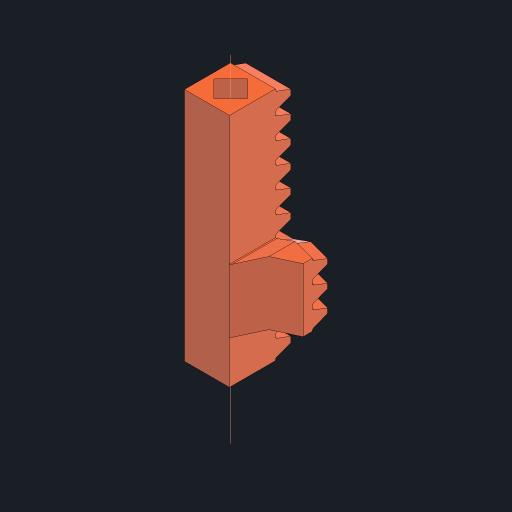
# Autodesk Inventor part: Rack V3
Saved by Autodesk Inventor 2023.2 (Build 272271030, 271C)
## iProperties
Created: 2023-11-19
Part Number: Rack V3
Material: Generic
Document SubType Name: Modeling
Designer: robpl
Density: 1 g/cm^3
Appearance: Smooth - Light Orange
Author: robpl
## iProperties of the stored document Rack_3DPrint.ipt
Created: 2023-11-27
Part Number: Rack_3DPrint
Material: Generic
Document SubType Name: Modeling
Designer: robpl
Density: 1 g/cm^3
Appearance: Default
Author: robpl
Autodesk Inventor part; units mm, degrees
ref_plane "YZ Plane" through (0, 0, 0) normal (1, 0, 0) x (0, 1, 0)
ref_plane "XZ Plane" through (0, 0, 0) normal (0, 1, 0) x (-1, 0, 0)
ref_plane "XY Plane" through (0, 0, 0) normal (0, 0, 1) x (1, 0, 0)
sketch "Sketch1" plane through (0, 0, 0) normal (0, 0, 1) x (1, 0, 0)
  line L0 (0, 0) -> (-12, 0)
  line L1 (-12, 0) -> (-12, 34.557519)
  line L2 (-12, 34.557519) -> (0, 34.557519)
  line L3 (0, 34.557519) -> (0, 0)
  dimension "d0" = 12
  dimension "d1" = 34.55752
  constraints: 8 end point, 2 parallel, 1 horizontal, 1 perpendicular
  measures "d0" distance of L1.end L2.end
  measures "d1" distance of L0.end L1.end
extrude "Extrusion1" add sketch "Sketch1" along normal blind 9
sketch "Sketch2" plane through (-12, 0, 0) normal (1, 0, 0) x (0, 0, -1)
  line L0 (0, 0) -> (0, 34.557519)
  line L1 (0, 34.557519) -> (-9, 34.557519)
  line L2 (-9, 0) -> (-9, 34.557519)
  line L3 (0, 0) -> (-9, 0)
  line L4 (0, 1.149368) -> (-2.25, 0.330435)
  line L5 (-2.25, 0.330435) -> (-2.25, -0.330435)
  line L6 (-2.25, -0.330435) -> (0, -1.149368)
  line L7 (0, -1.149368) -> (0, 1.149368)
  line L8 (-1, -0.785398) -> (-1, 0.785398)
  line L9 (0, 0) -> (-9, 0)
  arc A0 (-2.25, -0.064357) -> (-1.999968, -0.42144) centre (-1.87, -0.064357) ccw
  arc A1 (-1.999968, 0.42144) -> (-2.25, 0.064357) centre (-1.87, 0.064357) ccw
  point P0 (-2.25, 0)
  point P1 (0, 0)
  point P2 (-2.25, 0)
  dimension "d4" = 1
  dimension "d5" = 1.25
  dimension "d6" = 1.5708
  dimension "d7" = 70
  dimension "d17" = 0.38
  constraints: 10 end point, 8 point on line, 4 point on circle, 4 tangent, 3 vertical, 2 centre point, 1 equal length, 1 equal radius, 1 midpoint
  measures "d4" distance between parallel lines of L0 L8
  measures "d5" distance between parallel lines of L5 L8
  measures "d6" distance of L8.start L8.end
  measures "d7" angle of L6 L8
  measures "d17" radius of A0
sketch "Sketch3" plane through (0, 0, 0) normal (0, 0, -1) x (-1, 0, 0)
  line L0 (12, -1.149368) -> (12, 1.149368)
  line L1 (12, -1.149368) -> (5, -1.149368)
  line L2 (5, -1.149368) -> (2.5, -0.239443)
  line L3 (2.5, -0.239443) -> (0, -1.149368)
  point P0 (0, 0)
  dimension "d27" = 7
  dimension "d28" = 5
  dimension "d29" = 20
  constraints: 6 end point, 1 equal length, 1 horizontal, 1 point on line
  measures "d27" distance of L0.start L1.end
  measures "d28" distance of L1.end L3.end
  measures "d29" angle of L1 L2
sweep "Sweep1" cut profiles "Sketch2" path "Sketch3" path curves L1 L2 L3 contours L3 L8 L4 L0 | L7 L6 L8 L3 | L8 L6 A0 L5 L3 | L3 L5 A1 L4 L8
pattern_linear "Rectangular Pattern1" count 12 spacing 3.141593 along (0, 1, 0) of "Sweep1"
sketch "Sketch4" plane through (-12, 34.557519, 9) normal (0, 1, 0) x (1, 0, 0)
  line L0 (0, 6.75) -> (0, 0)
  line L1 (12, 0) -> (0, 0)
  line L2 (12, 6.750032) -> (12, 0)
  line L3 (3.3, 5.974874) -> (0.825126, 3.5)
  line L4 (0.825126, 3.5) -> (3.3, 1.025126)
  line L5 (3.3, 1.025126) -> (5.774874, 3.5)
  line L6 (5.774874, 3.5) -> (3.3, 5.974874)
  line L7 (3.3, 5.974874) -> (3.3, 1.025126) construction
  line L8 (0.825126, 3.5) -> (5.774874, 3.5) construction
  line L9 (0, 6.75) -> (0, 0)
  line L10 (0, 9) -> (7, 9)
  line L11 (10.970457, 7.000032) -> (9.5, 8.38181)
  line L12 (9.5, 8.38181) -> (8.029543, 7.000032)
  line L13 (6.985501, 6.75) -> (0, 6.75)
  ellipse E0 centre (12.014499, 7.13) end of major axis (10.903453, 7.13) minor radius 0.38 (10.970457, 7.000032) -> (12, 6.750032) ccw
  ellipse E1 centre (6.985501, 7.13) end of major axis (8.096547, 7.13) minor radius 0.38 (6.985501, 6.75) -> (8.029543, 7.000032) ccw
  point P0 (12, 9)
  point P1 (3.3, 3.5)
  point P2 (3.3, 3.5)
  point P3 (0, 3.375)
  dimension "d60" = 3.5
  dimension "d61" = 3.3
  dimension "d62" = 5.5
  constraints: 12 end point, 4 midpoint, 2 parallel, 2 perpendicular, 1 horizontal, 2 other
  measures "d60" distance between parallel lines of L3 L5
  measures "d61" distance between parallel lines of L0 L7
  measures "d62" distance between parallel lines of L10 L8
extrude "Extrusion8" cut sketch "Sketch4" against normal through all contours L6 L5 L4 L3
chamfer "Chamfer2" distance 5.4 angle 45 1 edges at (0, 17.2788, 9)
sketch "Sketch11" plane through (0, 0, 9) normal (0, 0, 1) x (1, 0, 0)
  line L0 (-12, 12.502014) -> (-5.191317, 12.502014)
  line L1 (-5.191317, 12.502014) -> (-2.5, 13.481573)
  line L2 (-2.5, 13.481573) -> (0, 12.571648)
  line L3 (-12, 22.055505) -> (-5.214012, 22.055505)
  line L4 (-5.214012, 22.055505) -> (-2.5, 23.043325)
  line L5 (-2.5, 23.043325) -> (0, 22.133399)
  line L6 (0, 34.557519) -> (-5.4, 34.557519)
  line L7 (-5.4, 34.557519) -> (-5.4, 0)
  line L8 (-5.4, 0) -> (0, 0)
  line L9 (0, 0) -> (0, 34.557519)
  line L10 (-5.4, 34.557519) -> (-5.4, 0)
  line L11 (-5.4, 34.557519) -> (-12, 34.557519)
  line L12 (-12, 34.557519) -> (-12, 0)
  line L13 (-12, 0) -> (-5.4, 0)
  line L14 (-3.970457, 0) -> (-5.014499, 0)
  line L15 (-5.4, 0) -> (-5.4, 34.557519)
  line L16 (0, 34.557519) -> (-5.4, 34.557519)
  line L17 (-2.5, 16.623166) -> (0, 15.71324)
  line L18 (-5.191317, 15.643607) -> (-2.5, 16.623166)
  line L19 (-12, 15.643607) -> (-5.191317, 15.643607)
  line L20 (-2.5, 7.335362) -> (0, 6.425436)
  line L21 (-5.214012, 6.347542) -> (-2.5, 7.335362)
  line L22 (-12, 6.347542) -> (-5.214012, 6.347542)
  point P0 (0, 22.133399)
  point P1 (-5.4, 22.055505)
  point P2 (-5.4, 12.502014)
  point P3 (0, 12.571648)
  point P4 (-5.4, 15.643607)
  point P5 (-5.4, 6.347542)
  dimension "d71" = 6.6
  constraints: 2 end point, 2 point on line, 1 vertical
  measures "d71" distance between parallel lines of L12 L15
extrude "Extrusion11" cut sketch "Sketch11" against normal through all contours L7 L3 L4 L5 L9 L17 L18 L19 | L22 L21 L20 L9 L8 L7 | L7 L6 L9 L5 L4 L3
equation "\"d5\" = 1.25 * d4"
equation "\"d6\" = 1.5708 * d4"
equation "\"d17\" = 0.38 * d4"
body "Solid1"
